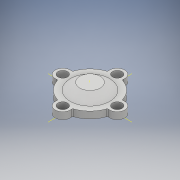
# Autodesk Inventor part: Деталь2
Saved by Autodesk Inventor 2018 (Build 220112000, 112)
## iProperties
Created: 2020-05-07
Part Number: Деталь2
Material: Типовые
Document SubType Name: Modeling
Designer: 2000
Density: 1 g/cm^3
Appearance: По умолчанию
Mass: 49.0412 g
Surface Area: 156.005 cm^2
Volume: 49.0412 cm^3
Author: 2000
Autodesk Inventor part; units mm, degrees
ref_plane "YZ Plane" through (0, 0, 0) normal (1, 0, 0) x (0, 1, 0)
ref_plane "XZ Plane" through (0, 0, 0) normal (0, 1, 0) x (-1, 0, 0)
ref_plane "XY Plane" through (0, 0, 0) normal (0, 0, 1) x (1, 0, 0)
sketch "Эскиз1" plane through (0, 0, 0) normal (0, 0, 1) x (1, 0, 0)
  arc A0 (-38.2043, 10.8524) -> (-38.2043, -10.8524) centre (-40, 0) ccw
  arc A1 (-10.8524, -38.2043) -> (10.8524, -38.2043) centre (0, -40) ccw
  arc A2 (10.8524, 38.2043) -> (-10.8524, 38.2043) centre (0, 40) ccw
  arc A3 (38.2043, -10.8524) -> (38.2043, 10.8524) centre (40, 0) ccw
  arc A4 (-38.2043, 10.8524) -> (-36.0537, 12.0056) centre (-37.8778, 12.8256) ccw
  arc A5 (-36.0537, -12.0056) -> (-38.2043, -10.8524) centre (-37.8778, -12.8256) ccw
  arc A6 (-10.8524, -38.2043) -> (-12.0056, -36.0537) centre (-12.8256, -37.8778) ccw
  arc A7 (12.0056, -36.0537) -> (10.8524, -38.2043) centre (12.8256, -37.8778) ccw
  arc A8 (38.2043, -10.8524) -> (36.0537, -12.0056) centre (37.8778, -12.8256) ccw
  arc A9 (36.0537, 12.0056) -> (38.2043, 10.8524) centre (37.8778, 12.8256) ccw
  arc A10 (10.8524, 38.2043) -> (12.0056, 36.0537) centre (12.8256, 37.8778) ccw
  arc A11 (-12.0056, 36.0537) -> (-10.8524, 38.2043) centre (-12.8256, 37.8778) ccw
  arc A12 (-12.0056, 36.0537) -> (-36.0537, 12.0056) centre (0, 0) ccw
  arc A13 (36.0537, 12.0056) -> (12.0056, 36.0537) centre (0, 0) ccw
  arc A14 (-36.0537, -12.0056) -> (-12.0056, -36.0537) centre (0, 0) ccw
  arc A15 (12.0056, -36.0537) -> (36.0537, -12.0056) centre (0, 0) ccw
  dimension "d87" = 22
  dimension "d88" = 22
  dimension "d89" = 22
  dimension "d90" = 22
  dimension "d91" = 40
  dimension "d92" = 40
  dimension "d93" = 40
  dimension "d94" = 40
  dimension "d95" = 4
  dimension "d96" = 4
  dimension "d97" = 4
  dimension "d98" = 4
  dimension "d99" = 4
  dimension "d100" = 4
  dimension "d101" = 4
  dimension "d102" = 4
  dimension "d103" = 38
  dimension "d104" = 38
  dimension "d105" = 38
  dimension "d106" = 38
  dimension "d107" = 37.8778
  dimension "d108" = 37.8778
  dimension "d109" = 37.8778
  dimension "d110" = 37.8778
  dimension "d111" = 37.8778
  dimension "d112" = 37.8778
  dimension "d113" = 37.8778
  dimension "d114" = 37.8778
  constraints: 32 point on circle, 16 centre point, 8 tangent, 2 horizontal alignment, 2 vertical alignment
  measures "d87" diameter of A0
  measures "d88" diameter of A1
  measures "d89" diameter of A3
  measures "d90" diameter of A2
  measures "d91" distance of A12.centre A2.centre
  measures "d92" distance of A1.centre A12.centre
  measures "d93" distance of A12.centre A0.centre
  measures "d94" distance of A12.centre A3.centre
  measures "d95" diameter of A5
  measures "d96" diameter of A4
  measures "d97" diameter of A11
  measures "d98" diameter of A10
  measures "d99" diameter of A9
  measures "d100" diameter of A8
  measures "d101" diameter of A7
  measures "d102" diameter of A6
  measures "d103" radius of A12
  measures "d104" radius of A14
  measures "d105" radius of A15
  measures "d106" radius of A13
  measures "d107" horizontal distance of A12.centre A8.centre
  measures "d108" vertical distance of A12.centre A7.centre
  measures "d109" vertical distance of A12.centre A6.centre
  measures "d110" horizontal distance of A12.centre A5.centre
  measures "d111" horizontal distance of A12.centre A4.centre
  measures "d112" vertical distance of A12.centre A11.centre
  measures "d113" vertical distance of A12.centre A10.centre
  measures "d114" horizontal distance of A12.centre A9.centre
extrude "Выдавливание1" add sketch "Эскиз1" along normal blind 20
sketch "Эскиз4" plane through (0, 0, 0) normal (0, 1, 0) x (-1, 0, 0)
  line L0 (0, 0) -> (29, 0)
  line L1 (0, 10) -> (15, 10)
  line L2 (15, 10) -> (29, 0)
  line L3 (0, 10) -> (0, 0)
  line L4 (11, 0) -> (-11, 0) projected
  line L5 (0, -4) -> (0, 24) projected
  point P0 (10.8524, 0)
  point P1 (-10.8524, 0)
  dimension "d115" = 29
  dimension "d116" = 15
  dimension "d117" = 10
  constraints: 8 end point, 2 horizontal, 1 perpendicular
  measures "d115" distance of L0.start L0.end
  measures "d116" distance of L1.start L1.end
  measures "d117" distance between parallel lines of L0 L1
revolve "Вращение4" cut sketch "Эскиз4" angle 360 about axis through (0, 0, -10) along (0, 0, 1)
sketch "Эскиз5" plane through (0, 0, 0) normal (0, 1, 0) x (-1, 0, 0)
  line L0 (-51, 0) -> (-51, 20) projected
  line L1 (-51, 10) -> (-29, 10)
  line L2 (-29, 10) -> (-15, 20)
  line L3 (-15, 20) -> (-51, 20)
  line L4 (-12.0056, 20) -> (-36.0537, 20) projected
  line L5 (-15, 10) -> (-29, 0) projected
  line L6 (-38.2043, 0) -> (-51, 0) projected
  line L7 (0, -4) -> (0, 24) projected
  point P0 (0, 0)
  dimension "d120" = 10
  dimension "d122" = 29
  constraints: 6 end point, 1 collinear, 1 horizontal, 1 midpoint, 1 parallel
  measures "d120" distance between parallel lines of L6 L1
  measures "d122" horizontal distance of point (0, 0) L1.end
revolve "Вращение5" cut sketch "Эскиз5" angle 360 about axis through (0, 0, -10) along (0, 0, 1)
sketch "Эскиз6" plane through (0, -40, 10) normal (0, 0, 1) x (1, 0, 0)
  circle A0 centre (0, 0) radius 7
  circle A1 centre (-40, 40) radius 7
  circle A2 centre (0, 80) radius 7
  circle A3 centre (40, 40) radius 7
  point P0 (0, 40)
  dimension "d125" = 40
  dimension "d126" = 40
  dimension "d127" = 40
  dimension "d128" = 40
  dimension "d129" = 14
  dimension "d130" = 14
  dimension "d131" = 14
  dimension "d132" = 14
  constraints: 4 centre point, 2 horizontal alignment, 2 vertical alignment
  measures "d125" distance of point (0, 40) A3.centre
  measures "d126" horizontal distance of A3.centre A0.centre
  measures "d127" distance of point (0, 40) A1.centre
  measures "d128" distance of point (0, 40) A2.centre
  measures "d129" diameter of A2
  measures "d130" diameter of A1
  measures "d131" diameter of A0
  measures "d132" diameter of A3
hole "Отверстие1" at (0, -40, 10) at (-40, 0, 10) at (40, 0, 10) at (0, 40, 10) direction (0, 0, -1) diameter 14 depth 10
